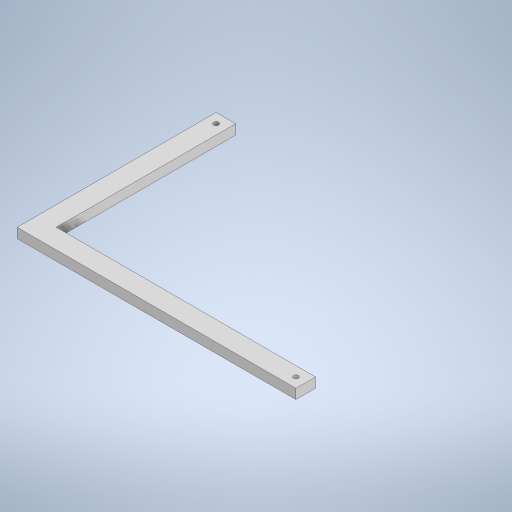
# Autodesk Inventor part: ArmRest(H)
Saved by Autodesk Inventor 2023 (Build 270158030, 158C)
## iProperties
Created: 2023-03-04
Part Number: ArmRest(H)
Material: Generic
Document SubType Name: Modeling
Designer: mpino
Density: 1 g/cm^3
Appearance: Default
Author: mpino
Autodesk Inventor part; units mm, degrees
ref_plane "YZ Plane" through (0, 0, 0) normal (1, 0, 0) x (0, 1, 0)
ref_plane "XZ Plane" through (0, 0, 0) normal (0, 1, 0) x (-1, 0, 0)
ref_plane "XY Plane" through (0, 0, 0) normal (0, 0, 1) x (1, 0, 0)
sketch "Sketch7" plane through (0, 0, 0) normal (1, 0, 0) x (0, 1, 0)
  line L0 (6.35, 12.7) -> (-6.35, 12.7)
  line L1 (-6.35, 12.7) -> (-6.35, -12.7)
  line L2 (-6.35, -12.7) -> (6.35, -12.7)
  line L3 (6.35, -12.7) -> (6.35, 12.7)
  line L4 (6.35, 12.7) -> (-6.35, -12.7) construction
  line L5 (-6.35, 12.7) -> (6.35, -12.7) construction
  point P0 (0, 0)
  dimension "d30" = 12.7
  dimension "d31" = 25.4
  constraints: 12 end point, 2 midpoint, 2 parallel, 1 horizontal, 1 perpendicular
  measures "d30" distance of L2.end L1.end
  measures "d31" distance of L1.end L0.end
sketch "Sketch9" plane through (0, 0, 0) normal (0, 1, 0) x (-1, 0, 0)
  line L0 (0, 0) -> (348.0816, 0)
  line L1 (348.0816, 0) -> (348.0816, -244.729)
  dimension "d34" = 244.729
  dimension "d35" = 348.0816
  constraints: 4 end point, 1 horizontal, 1 perpendicular
  measures "d34" distance of L0.end L1.end
  measures "d35" distance from line of L0.start L1
sweep "Sweep2" add profiles "Sketch7" path "Sketch9"
sketch "Sketch10" plane through (0, 6.35, 12.7) normal (0, 1, 0) x (1, 0, 0)
  line L0 (0, 0) -> (0, 25.4) projected
  line L1 (0, 25.4) -> (-335.3816, 25.4) projected
  line L2 (0, 0) -> (-25.4, 0)
  line L3 (-25.4, 0) -> (-25.4, 25.4)
  line L4 (-25.4, 25.4) -> (0, 25.4)
  line L5 (0, 25.4) -> (0, 0)
  circle A0 centre (-12.7, 12.7) radius 3.175
  line L6 (-335.3816, 257.429) -> (-360.7816, 257.429) projected
  line L7 (-360.7816, 0) -> (-360.7816, 257.429) projected
  line L8 (-335.3816, 257.429) -> (-360.7816, 257.429)
  line L9 (-360.7816, 257.429) -> (-360.7816, 232.029)
  line L10 (-360.7816, 232.029) -> (-335.3816, 232.029)
  line L11 (-335.3816, 232.029) -> (-335.3816, 257.429)
  circle A1 centre (-348.0816, 244.729) radius 3.175
  point P0 (0, 12.7)
  point P1 (-25.4, 12.7)
  point P2 (-12.7, 25.4)
  dimension "d38" = 25.4
  dimension "d39" = 6.35
  dimension "d40" = 12.7
  dimension "d41" = 12.7
  dimension "d42" = 25.4
  dimension "d43" = 6.35
  dimension "d44" = 12.7
  dimension "d45" = 12.7
  constraints: 16 end point, 4 parallel, 2 centre point, 2 horizontal, 2 midpoint, 2 perpendicular, 2 point on line
  measures "d38" distance of L3.end L4.end
  measures "d39" diameter of A0
  measures "d40" distance of point (-25.4, 12.7) A0.centre
  measures "d41" distance of point (-12.7, 25.4) A0.centre
  measures "d42" distance of L9.end L8.end
  measures "d43" diameter of A1
  measures "d44" distance from line of L10 A1.centre
  measures "d45" distance from line of L7 A1.centre
extrude "Extrusion4" cut sketch "Sketch10" against normal blind 25.4 contours A0 | A1
body "Solid3"
